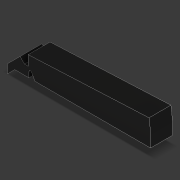
# Autodesk Inventor part: black_key
Saved by Autodesk Inventor 2020.2 (Build 242310000, 310)
## iProperties
Created: 2020-07-05
Part Number: black_key
Material: Black ABS
Document SubType Name: Modeling
Designer: isaac
Density: 1.06 g/cm^3
Appearance: Smooth - White(1)
Author: isaac
Autodesk Inventor part; units mm, degrees
ref_plane "YZ Plane" through (0, 0, 0) normal (1, 0, 0) x (0, 1, 0)
ref_plane "XZ Plane" through (0, 0, 0) normal (0, 1, 0) x (-1, 0, 0)
ref_plane "XY Plane" through (0, 0, 0) normal (0, 0, 1) x (1, 0, 0)
sketch "Sketch1" plane through (0, 0, 0) normal (1, 0, 0) x (0, 1, 0)
  line L0 (-2.5263, 2.1514) -> (-2.5263, 54.9419)
  arc A0 (9.0738, 54.2463) -> (-2.5263, 54.9419) centre (0, 0) ccw
  line L1 (9.0738, 54.2463) -> (6.4541, -0.9785)
  line L2 (-2.5263, 2.1514) -> (0.3, 0.5196)
  arc A1 (0, -0.6) -> (0.3, 0.5196) centre (0, 0) ccw
  line L3 (0, -0.6) -> (-2.5263, -0.6)
  line L4 (-2.5263, -0.6) -> (-2.5263, -7.0839)
  line L5 (-2.5263, -7.0839) -> (-5.8882, -10.4459)
  line L6 (-5.8882, -10.4459) -> (-1.8882, -10.4459)
  line L7 (6.4541, -0.9785) -> (1.8773, -0.9785)
  line L8 (1.8773, -2.6803) -> (3.8773, -4.6803)
  line L9 (3.8773, -4.6803) -> (-1.8882, -10.4459)
  line L10 (1.8773, -2.6803) -> (1.8773, -0.9785)
  dimension "d0" = 0.6
  dimension "d2" = 45
  dimension "d3" = 2
  dimension "d4" = 55
  dimension "d7" = 60
  constraints: 22 end point, 4 point on circle, 3 horizontal, 3 vertical, 2 centre point, 2 coincident, 2 tangent, 1 parallel, 1 perpendicular, 1 point on line
  measures "d0" radius of A1
  measures "d2" angle of L4 L5
  measures "d3" distance from line of L8.end L10
  measures "d4" radius of A0
  measures "d7" angle of L2 L0
extrude "Extrusion1" add sketch "Sketch1" along normal mid plane 10
equation "\"d0\" = hingeSocketRad"
equation "\"d4\" = blackKeyLength"
equation "\"d7\" = hingeOverhangAngle"
equation "\"hingeSocketRad\" = 0.6"
equation "\"blackKeyLength\" = 55"
equation "\"hingeOverhangAngle\" = 60deg"
body "Solid1"
